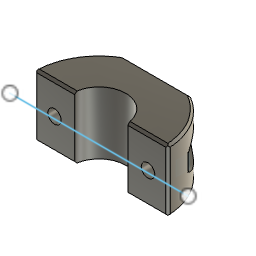
リードマグネットマウント (Autodesk Fusion 360 design; units mm, degrees)
Autodesk Fusion 360 part; units mm, degrees
note: some values were not read from the file. Set by a fixed rule: which sketch regions a step uses.
sketch "スケッチ2" plane through (0, 0, 0) normal (0, 0, 1) x (1, 0, 0)
  line L0 (0, 0.5) -> (0, -0.5)
  arc A0 (-7.4833, 13) -> (-14.9917, 0.4998) centre (0, 0) ccw
  line L1 (-14.9917, 0.4998) -> (-5.9791, 0.4998)
  line L2 (5.9791, 0.4998) -> (14.9917, 0.4998)
  arc A1 (5.9791, 0.4998) -> (-5.9791, 0.4998) centre (0, 0) ccw
  arc A2 (14.9917, 0.4998) -> (7.4833, 13) centre (0, 0) ccw
  line L3 (0, 13) -> (7.4833, 13)
  line L4 (-7.4833, 13) -> (0, 13)
  constraint vertical L0
  constraint perpendicular L0 L1
  constraint collinear L1 L2
extrude "押し出し1" add sketch "スケッチ2" along normal blind 14
sketch "スケッチ4" plane through (0, 13, 0) normal (0, 1, 0) x (-1, 0, 0)
  line L0 (-7.4833, 0) -> (7.4833, 0)
  line L1 (7.4833, 0) -> (7.4833, 14)
  line L2 (7.4833, 14) -> (-7.4833, 14)
  line L3 (-7.4833, 14) -> (-7.4833, 0)
  circle A0 centre (0, 7) radius 6
  dimension "d7" = 12
  measures "d7" diameter of A0
extrude "押し出し2" cut sketch "スケッチ4" against normal blind 1 contours A0
sketch "スケッチ5" plane through (0, 0, 0) normal (0, 1, 0) x (1, 0, 0)
  line L0 (0, 1) -> (0, -15)
  line L1 (15, -7) -> (10.5, -7)
  circle A0 centre (10.5, -7) radius 1.5
  circle A1 centre (-10.5, -7) radius 1.5
  dimension "d10" = 4.5
  constraint vertical L0
  constraint perpendicular L0 L1
  constraint coincident L1.end A0.centre
  constraint symmetric L0 A0 A1
  measures "d10" distance of L1.start L1.end
extrude "押し出し3" cut sketch "スケッチ5" along normal blind 13
sketch "スケッチ6" plane through (0, 13, 0) normal (0, 1, 0) x (-1, 0, 0)
  circle A0 centre (0, 7) radius 6
  line L0 (-7.4833, 0) -> (7.4833, 0)
  line L1 (7.4833, 0) -> (7.4833, 14)
  line L2 (7.4833, 14) -> (-7.4833, 14)
  line L3 (-7.4833, 14) -> (-7.4833, 0)
  circle A1 centre (10.5, 7) radius 3.5
  line L4 (-7.7, 8.6166) -> (-10.5, 10.2332)
  line L5 (-10.5, 10.2332) -> (-13.3, 8.6166)
  line L6 (-13.3, 8.6166) -> (-13.3, 5.3834)
  line L7 (-13.3, 5.3834) -> (-10.5, 3.7668)
  line L8 (-10.5, 3.7668) -> (-7.7, 5.3834)
  line L9 (-7.7, 5.3834) -> (-7.7, 8.6166)
  point P0 (10.5, 7)
  point P1 (-10.5, 7)
  point P2 (-10.5, 7)
  constraint coincident P0 A1.centre
extrude "押し出し4" cut sketch "スケッチ6" against normal blind 9 contours L1 A1 | L1 A1 | L4 L5 L6 L7 L8 L9
sketch "スケッチ7" plane through (13.3, 0, 0) normal (-1, 0, 0) x (0, -1, 0)
  line L0 (-6.9361, 8.6166) -> (-6.9361, 5.3834)
  line L1 (-6.9361, 5.3834) -> (-4, 5.3834)
  line L2 (-4, 5.3834) -> (-4, 8.6166)
  line L3 (-4, 8.6166) -> (-6.9361, 8.6166)
chamfer "面取り1" distance 0.5 angle 45 8 edges at (0, 13, 0) (-12.8586, 7.7237, 0) (-14.9917, 0.4998, 7) (-12.8586, 7.7237, 14) (0, 13, 14) (12.8586, 7.7237, 14) (12.8586, 7.7237, 0) (14.9917, 0.4998, 7)
sketch "スケッチ8" plane through (0, 13, 0) normal (0, 1, 0) x (-1, 0, 0)
  circle A0 centre (0, 7) radius 6
  line L0 (7.4833, 13.5) -> (-7.4833, 13.5)
  line L1 (-7.4833, 13.5) -> (-7.4833, 0.5)
  line L2 (-7.4833, 0.5) -> (7.4833, 0.5)
  line L3 (7.4833, 0.5) -> (7.4833, 5.2253)
  arc A1 (7.4833, 8.7747) -> (7.4833, 5.2253) centre (10.5, 7) ccw
  line L4 (7.4833, 8.7747) -> (7.4833, 13.5)
  circle A2 centre (-10.5, 7) radius 3.5
  point P0 (-10.5, 7)
  dimension "d18" = 7
  constraint coincident P0 A2.centre
  measures "d18" diameter of A2
extrude "押し出し5" cut sketch "スケッチ8" against normal blind 6.5 contours L1 A2 | L1 A2
chamfer "面取り2" distance 0.5 angle 45 4 edges at (-10.2353, 0.4998, 14) (-10.2353, 0.4998, 0) (10.2353, 0.4998, 0) (10.2353, 0.4998, 14)
sketch "スケッチ9" plane through (0, 0, 0) normal (0, 1, 0) x (1, 0, 0)
  line L0 (20, -7) -> (-20, -7)
  constraint horizontal L0
